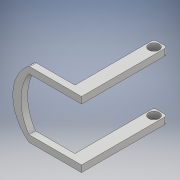
# Autodesk Inventor part: Mandibula
Saved by Autodesk Inventor 2017 SP1 (Build 210196100, 196)
## iProperties
Part Number: Mandibula
Material: Genérico
Document SubType Name: Modeling
Designer: Juan
Density: 1 g/cm^3
Appearance: Valor por defecto
Author: Juan
Autodesk Inventor part; units mm, degrees
ref_plane "YZ Plane" through (0, 0, 0) normal (1, 0, 0) x (0, 1, 0)
ref_plane "XZ Plane" through (0, 0, 0) normal (0, 1, 0) x (-1, 0, 0)
ref_plane "XY Plane" through (0, 0, 0) normal (0, 0, 1) x (1, 0, 0)
sketch "Boceto1" plane through (0, 0, 0) normal (0, 1, 0) x (-1, 0, 0)
  line L0 (1.3392, 10.6007) -> (1.3392, 5.6007)
  line L1 (1.3392, 5.6007) -> (41.3392, 5.6007)
  line L2 (1.3392, 10.6007) -> (41.3392, 10.6007)
  arc A0 (41.3392, -34.3993) -> (41.3392, 5.6007) centre (10.5353, -14.3993) ccw
  line L3 (41.3392, -34.3993) -> (1.3392, -34.3993)
  line L4 (1.3392, -34.3993) -> (1.3392, -39.3993)
  line L5 (1.3392, -39.3993) -> (41.3392, -39.3993)
  arc A1 (41.3392, -39.3993) -> (41.3392, 10.6007) centre (21.6641, -14.3993) ccw
  point P0 (0, 0)
  dimension "d0" = 5
  dimension "d1" = 40
  dimension "d2" = 40
  dimension "d3" = 5
  constraints: 12 end point, 4 point on circle, 3 perpendicular, 2 centre point, 2 horizontal, 1 vertical
  measures "d0" distance of L0.start L0.end
  measures "d1" distance of L0.end L1.end
  measures "d2" distance of L1.end L3.start
  measures "d3" distance of L3.end L4.end
extrude "Extrusión1" add sketch "Boceto1" along normal blind 5
ref_plane "Plano de trabajo1" through (0, 5, 0) normal (0, 1, 0) x (1, 0, 0)
sketch "Boceto2" plane through (0, 5, 0) normal (0, 1, 0) x (1, 0, 0)
  line L0 (-1.3392, 34.3993) -> (-1.3392, 39.3993) projected
  line L1 (-1.3392, 39.3993) -> (-11.3392, 39.3993)
  line L2 (-11.3392, 39.3993) -> (-11.3392, 34.3993)
  line L3 (-11.3392, 34.3993) -> (-1.3392, 34.3993)
  line L4 (-1.3392, 34.3993) -> (-1.3392, 39.3993)
  line L5 (-1.3392, -10.6007) -> (-1.3392, -5.6007) projected
  line L6 (-1.3392, -5.6007) -> (-11.3392, -5.6007)
  line L7 (-11.3392, -5.6007) -> (-11.3392, -10.6007)
  line L8 (-11.3392, -10.6007) -> (-1.3392, -10.6007)
  line L9 (-1.3392, -10.6007) -> (-1.3392, -5.6007)
  point P0 (0, 0)
  dimension "d7" = 10
  dimension "d8" = 10
  constraints: 16 end point, 4 parallel, 2 horizontal, 2 perpendicular
  measures "d7" distance of L3.end L2.end
  measures "d8" distance of L8.end L7.end
extrude "Extrusión2" add sketch "Boceto2" along normal blind 45
ref_plane "Plano de trabajo2" through (0, 50, 0) normal (0, 1, 0) x (1, 0, 0)
ref_plane "Plano de trabajo3" through (0, 50, 0) normal (0, 1, 0) x (1, 0, 0)
sketch "Boceto3" plane through (0, 50, 0) normal (0, 1, 0) x (1, 0, 0)
  line L0 (-1.3392, -10.6007) -> (-1.3392, -5.6007) projected
  line L1 (-11.3392, -10.6007) -> (-1.3392, -10.6007)
  line L2 (-1.3392, -10.6007) -> (-1.3392, -5.6007)
  line L3 (-1.3392, -5.6007) -> (-11.3392, -5.6007)
  line L4 (-11.3392, -5.6007) -> (-11.3392, -10.6007)
  line L5 (-11.3392, 39.3993) -> (-11.3392, 34.3993) projected
  line L6 (-11.3392, 39.3993) -> (-1.3392, 39.3993)
  line L7 (-1.3392, 39.3993) -> (-1.3392, 34.3993)
  line L8 (-1.3392, 34.3993) -> (-11.3392, 34.3993)
  line L9 (-11.3392, 34.3993) -> (-11.3392, 39.3993)
  point P0 (0, 0)
  constraints: 16 end point, 4 parallel, 2 horizontal, 2 perpendicular
extrude "Extrusión3" add sketch "Boceto3" along normal blind 15
ref_plane "Plano de trabajo4" through (-41.3392, 0, 10.6007) normal (0, 0, 1) x (1, 0, 0)
sketch "Boceto4" plane through (-41.3392, 0, 10.6007) normal (0, 0, 1) x (1, 0, 0)
  line L0 (30, 65) -> (40, 65) construction
  line L1 (35, 65) -> (35, 60) construction
  point P0 (41.3392, 0)
  dimension "d17" = 5
  constraints: 2 end point, 1 midpoint, 1 vertical
  measures "d17" distance of L1.start L1.end
hole "Agujero1" at (-6.3392, 60, 10.6007) direction (0, 0, -1) diameter 8 end through all
fillet "Empalme2" radius 2 4 edges at (-1.3392, 65, -36.8993) (-1.3392, 65, 8.1007) (-11.3392, 65, 8.1007) (-11.3392, 65, -36.8993)
fillet "Empalme3" radius 2 1 edges at (-41.3392, 2.5, -39.3993)
fillet "Empalme4" radius 2 1 edges at (-41.3392, 2.5, 10.6007)
equation "\"d8\" = d7"
